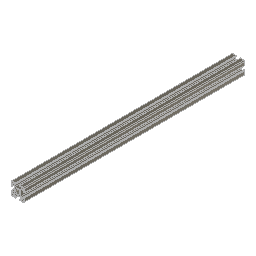
Профиль 3030 500mm (Autodesk Fusion 360 design; units mm, degrees)
Autodesk Fusion 360 part; units mm, degrees
sketch "Sketch1" plane through (0, 0, 0) normal (0, 1, 0) x (1, 0, 0)
  line L0 (6.0101, -7) -> (-6.0101, -7)
  line L1 (-8.1, -12.8) -> (-8.1, -9.0899)
  line L2 (-6.0101, -7) -> (-8.1, -9.0899)
  line L3 (-4.1, -14.2) -> (-4.9, -14.2)
  line L4 (-4.9, -14.2) -> (-4.9, -15)
  line L5 (-4.1, -14.2) -> (-4.1, -12.8)
  line L6 (-13, -15) -> (-4.9, -15)
  line L7 (-8.1, -12.8) -> (-4.1, -12.8)
  line L8 (6.0101, -7) -> (8.1, -9.0899)
  line L9 (8.1, -12.8) -> (8.1, -9.0899)
  line L10 (8.1, -12.8) -> (4.1, -12.8)
  line L11 (4.1, -14.2) -> (4.1, -12.8)
  line L12 (4.1, -14.2) -> (4.9, -14.2)
  line L13 (4.9, -14.2) -> (4.9, -15)
  line L14 (13, -15) -> (4.9, -15)
  line L15 (14.2, -4.1) -> (14.2, -4.9)
  line L16 (12.8, -8.1) -> (9.0899, -8.1)
  line L17 (15, -13) -> (15, -4.9)
  line L18 (7, 6.0101) -> (9.0899, 8.1)
  line L19 (7, 6.0101) -> (7, -6.0101)
  line L20 (14.2, 4.9) -> (15, 4.9)
  line L21 (7, -6.0101) -> (9.0899, -8.1)
  line L22 (14.2, -4.1) -> (12.8, -4.1)
  line L23 (14.2, 4.1) -> (12.8, 4.1)
  line L24 (15, 13) -> (15, 4.9)
  line L25 (14.2, -4.9) -> (15, -4.9)
  line L26 (12.8, 8.1) -> (9.0899, 8.1)
  line L27 (12.8, 8.1) -> (12.8, 4.1)
  line L28 (12.8, -8.1) -> (12.8, -4.1)
  line L29 (14.2, 4.1) -> (14.2, 4.9)
  line L30 (4.1, 14.2) -> (4.9, 14.2)
  line L31 (8.1, 12.8) -> (8.1, 9.0899)
  line L32 (13, 15) -> (4.9, 15)
  line L33 (-6.0101, 7) -> (-8.1, 9.0899)
  line L34 (-6.0101, 7) -> (6.0101, 7)
  line L35 (-4.9, 14.2) -> (-4.9, 15)
  line L36 (6.0101, 7) -> (8.1, 9.0899)
  line L37 (4.1, 14.2) -> (4.1, 12.8)
  line L38 (-4.1, 14.2) -> (-4.1, 12.8)
  line L39 (-13, 15) -> (-4.9, 15)
  line L40 (4.9, 14.2) -> (4.9, 15)
  line L41 (-8.1, 12.8) -> (-8.1, 9.0899)
  line L42 (-8.1, 12.8) -> (-4.1, 12.8)
  line L43 (8.1, 12.8) -> (4.1, 12.8)
  line L44 (-4.1, 14.2) -> (-4.9, 14.2)
  line L45 (-14.2, 4.1) -> (-14.2, 4.9)
  line L46 (-12.8, 8.1) -> (-9.0899, 8.1)
  line L47 (-15, 13) -> (-15, 4.9)
  line L48 (-7, -6.0101) -> (-9.0899, -8.1)
  line L49 (-7, -6.0101) -> (-7, 6.0101)
  line L50 (-14.2, -4.9) -> (-15, -4.9)
  line L51 (-7, 6.0101) -> (-9.0899, 8.1)
  line L52 (-14.2, 4.1) -> (-12.8, 4.1)
  line L53 (-14.2, -4.1) -> (-12.8, -4.1)
  line L54 (-15, -13) -> (-15, -4.9)
  line L55 (-14.2, 4.9) -> (-15, 4.9)
  line L56 (-12.8, -8.1) -> (-9.0899, -8.1)
  line L57 (-12.8, -8.1) -> (-12.8, -4.1)
  line L58 (-12.8, 8.1) -> (-12.8, 4.1)
  line L59 (-14.2, -4.1) -> (-14.2, -4.9)
  circle A0 centre (0, 0) radius 5
  circle A1 centre (-11.55, -11.55) radius 2.25
  circle A2 centre (11.55, -11.55) radius 2.25
  circle A3 centre (11.55, 11.55) radius 2.25
  circle A4 centre (-11.55, 11.55) radius 2.25
  arc A5 (-15, -13) -> (-13, -15) centre (-13, -13) ccw
  arc A6 (13, -15) -> (15, -13) centre (13, -13) ccw
  arc A7 (15, 13) -> (13, 15) centre (13, 13) ccw
  arc A8 (-13, 15) -> (-15, 13) centre (-13, 13) ccw
  dimension "d17" = 10
  dimension "d22" = 4.5
  dimension "d24" = 360
  dimension "d25" = 2
  constraint coincident A0.centre origin
  constraint tangent L54 A5
  constraint tangent L6 A5
  constraint tangent L14 A6
  constraint tangent L17 A6
  constraint equal A5 A6
  constraint tangent L24 A7
  constraint tangent L32 A7
  constraint equal A5 A7
  constraint tangent L39 A8
  constraint tangent L47 A8
  constraint equal A5 A8
  measures "d17" diameter of A0
  measures "d22" diameter of A1
  measures "d25" radius of A5
extrude "Extrude1" add sketch "Sketch1" along normal blind 500
